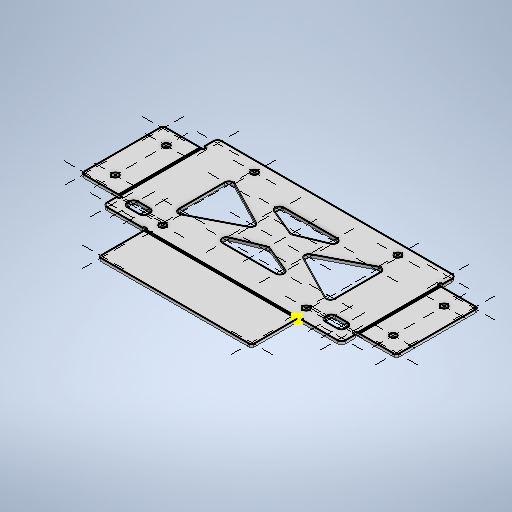
# Autodesk Inventor part: body_back_frame
Saved by Autodesk Inventor 2026.1 (Build 301233000, 233)
## iProperties
Created: 2025-08-22
Part Number: body_back_frame
Material: Generic
Document SubType Name: Modeling
Designer: chris
Density: 1 g/cm^3
Appearance: Default
Author: chris
Autodesk Inventor part; units mm, degrees
ref_plane "YZ Plane" through (0, 0, 0) normal (1, 0, 0) x (0, 1, 0)
ref_plane "XZ Plane" through (0, 0, 0) normal (0, 1, 0) x (-1, 0, 0)
ref_plane "XY Plane" through (0, 0, 0) normal (0, 0, 1) x (1, 0, 0)
sketch "Sketch1" plane through (0, 0, 0) normal (0, 1, 0) x (-1, 0, 0)
  line L0 (75, -0.4496) -> (0, -0.4496)
  line L1 (-21.1396, -9.0893) -> (-21.1396, -49.0893)
  line L2 (96.1396, -49.0893) -> (96.1396, -9.0893)
  circle A0 centre (72.69, -51.8993) radius 1.55
  circle A1 centre (2.31, -51.8993) radius 1.55
  circle A2 centre (72.69, -6.8993) radius 1.55
  circle A3 centre (2.31, -6.8993) radius 1.55
  arc A4 (-6, -7.8993) -> (-8, -5.8993) centre (-8, -7.8993) ccw
  line L3 (-14, -5.8993) -> (-8, -5.8993)
  arc A5 (-8, -10.8993) -> (-6, -8.8993) centre (-8, -8.8993) ccw
  line L4 (-6, -7.8993) -> (-6, -8.8993)
  arc A6 (-16, -8.8993) -> (-14, -10.8993) centre (-14, -8.8993) ccw
  line L5 (-16, -8.8993) -> (-16, -7.8993)
  arc A7 (-14, -5.8993) -> (-16, -7.8993) centre (-14, -7.8993) ccw
  arc A8 (89, -10.8993) -> (91, -8.8993) centre (89, -8.8993) ccw
  line L6 (91, -7.8993) -> (91, -8.8993)
  arc A9 (81, -8.8993) -> (83, -10.8993) centre (83, -8.8993) ccw
  line L7 (81, -8.8993) -> (81, -7.8993)
  arc A10 (91, -7.8993) -> (89, -5.8993) centre (89, -7.8993) ccw
  line L8 (83, -5.8993) -> (89, -5.8993)
  arc A11 (83, -5.8993) -> (81, -7.8993) centre (83, -7.8993) ccw
  arc A12 (2.2291, -16.0132) -> (-0.69, -17.7895) centre (1.31, -17.7895) ccw
  line L9 (-0.69, -40.389) -> (-0.69, -17.7895)
  arc A13 (24.0671, -30.8656) -> (24.0671, -27.313) centre (23.148, -29.0893) ccw
  line L10 (2.2291, -16.0132) -> (24.0671, -27.313)
  arc A14 (-0.69, -40.389) -> (2.2291, -42.1653) centre (1.31, -40.389) ccw
  line L11 (24.0671, -30.8656) -> (2.2291, -42.1653)
  arc A15 (23.6713, -40.2421) -> (24.4379, -44.0893) centre (24.4379, -42.0893) ccw
  line L12 (23.6713, -40.2421) -> (36.7334, -34.821)
  arc A16 (50.5621, -44.0893) -> (51.3287, -40.2421) centre (50.5621, -42.0893) ccw
  line L13 (38.2666, -34.821) -> (51.3287, -40.2421)
  arc A17 (38.2666, -34.821) -> (36.7334, -34.821) centre (37.5, -36.6682) ccw
  arc A18 (50.9329, -27.313) -> (50.9329, -30.8656) centre (51.852, -29.0893) ccw
  line L14 (50.9329, -27.313) -> (72.7709, -16.0132)
  arc A19 (75.69, -17.7895) -> (72.7709, -16.0132) centre (73.69, -17.7895) ccw
  line L15 (75.69, -17.7895) -> (75.69, -40.389)
  arc A20 (72.7709, -42.1653) -> (75.69, -40.389) centre (73.69, -40.389) ccw
  arc A21 (36.7334, -23.3576) -> (38.2666, -23.3576) centre (37.5, -21.5104) ccw
  line L16 (51.3287, -17.9365) -> (38.2666, -23.3576)
  arc A22 (51.3287, -17.9365) -> (50.5621, -14.0893) centre (50.5621, -16.0893) ccw
  line L17 (24.4379, -14.0893) -> (50.5621, -14.0893)
  arc A23 (24.4379, -14.0893) -> (23.6713, -17.9365) centre (24.4379, -16.0893) ccw
  line L18 (36.7334, -23.3576) -> (23.6713, -17.9365)
  line L19 (89, -10.8993) -> (83, -10.8993)
  line L20 (-8, -10.8993) -> (-14, -10.8993)
  circle A24 centre (-30.6843, -41.5893) radius 1.55
  circle A25 centre (105.6843, -41.5893) radius 1.55
  circle A26 centre (-30.6843, -16.5893) radius 1.55
  circle A27 centre (105.6843, -16.5893) radius 1.55
  line L21 (72.7709, -42.1653) -> (50.9329, -30.8656)
  line L22 (50.5621, -44.0893) -> (24.4379, -44.0893)
  arc A28 (-21, -55.0893) -> (-19, -57.0893) centre (-19, -55.0893) ccw
  line L23 (-19, -57.0893) -> (94, -57.0893)
  arc A29 (94, -57.0893) -> (96, -55.0893) centre (94, -55.0893) ccw
  line L24 (96, -50.5893) -> (96, -55.0893)
  arc A30 (96, -2.8993) -> (94, -0.8993) centre (94, -2.8993) ccw
  line L25 (94, -0.8993) -> (76.5, -0.8993)
  arc A31 (-19, -0.8993) -> (-21, -2.8993) centre (-19, -2.8993) ccw
  line L26 (-1.5, -0.8993) -> (-19, -0.8993)
  line L27 (96, -2.8993) -> (96, -7.5893)
  line L28 (-1.5, -1.6493) -> (-1.5, -0.8993)
  arc A32 (113.7793, -49.0893) -> (114.7793, -48.0893) centre (113.7793, -48.0893) ccw
  line L29 (114.7793, -10.0893) -> (114.7793, -48.0893)
  arc A33 (114.7793, -10.0893) -> (113.7793, -9.0893) centre (113.7793, -10.0893) ccw
  arc A34 (75, 21.19) -> (74, 22.19) centre (74, 21.19) ccw
  line L30 (1, 22.19) -> (74, 22.19)
  arc A35 (-39.7793, -48.0893) -> (-38.7793, -49.0893) centre (-38.7793, -48.0893) ccw
  arc A36 (-38.7793, -9.0893) -> (-39.7793, -10.0893) centre (-38.7793, -10.0893) ccw
  line L31 (-38.7793, -9.0893) -> (-19.94, -9.0893)
  arc A37 (1, 22.19) -> (0, 21.19) centre (1, 21.19) ccw
  line L32 (113.7793, -49.0893) -> (94.94, -49.0893)
  line L33 (-39.7793, -48.0893) -> (-39.7793, -10.0893)
  line L34 (96, -50.5893) -> (94.94, -50.5893)
  line L35 (94.94, -50.5893) -> (94.94, -49.0893)
  line L36 (94.94, -7.5893) -> (96, -7.5893)
  line L37 (94.94, -9.0893) -> (113.7793, -9.0893)
  line L38 (94.94, -9.0893) -> (94.94, -7.5893)
  line L39 (-21, -7.5893) -> (-19.94, -7.5893)
  line L40 (-19.94, -7.5893) -> (-19.94, -9.0893)
  line L41 (-21, -7.5893) -> (-21, -2.8993)
  line L42 (-19.94, -50.5893) -> (-21, -50.5893)
  line L43 (-19.94, -49.0893) -> (-38.7793, -49.0893)
  line L44 (-19.94, -49.0893) -> (-19.94, -50.5893)
  line L45 (-21, -55.0893) -> (-21, -50.5893)
  line L46 (75, 21.19) -> (75, -1.6493)
  line L47 (0, -1.6493) -> (0, 21.19)
  line L48 (0, -1.6493) -> (-1.5, -1.6493)
  line L49 (76.5, -0.8993) -> (76.5, -1.6493)
  line L50 (76.5, -1.6493) -> (75, -1.6493)
  line L51 (96.5893, -9.0893) -> (96.5893, -49.0893)
  line L52 (-21.5893, -49.0893) -> (-21.5893, -9.0893)
  line L53 (95.69, -49.0893) -> (95.69, -9.0893)
  line L54 (-20.69, -9.0893) -> (-20.69, -49.0893)
  line L55 (75, -0.8993) -> (0, -0.8993)
  line L56 (0, 0) -> (75, 0)
  constraints: 114 end point, 74 tangent, 60 point on circle, 38 centre point, 35 equal radius, 26 vertical, 24 parallel, 23 horizontal, 22 perpendicular, 18 point on line, 181 other
extrude "Extrusion1" add sketch "Sketch1" against normal blind 1.5
body "Solid1"
